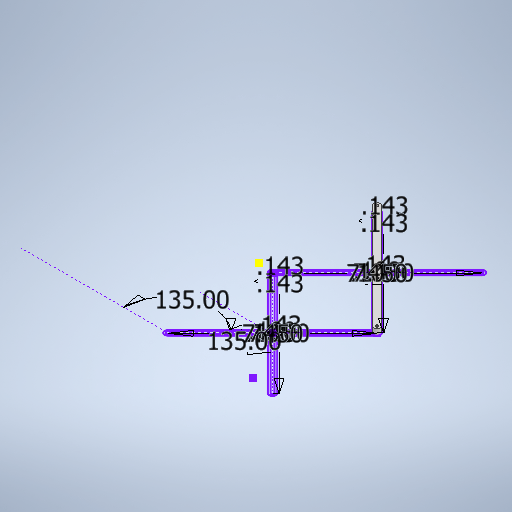
# Autodesk Inventor part: Arm
Saved by Autodesk Inventor 2025.1 (Build 291241000, 241)
## iProperties
Created: 2025-10-25
Part Number: Arm
Material: Generic
Document SubType Name: Modeling
Designer: benja
Density: 1 g/cm^3
Appearance: Default
Author: benja
Autodesk Inventor part; units mm, degrees
ref_plane "YZ Plane" through (0, 0, 0) normal (1, 0, 0) x (0, 1, 0)
ref_plane "XZ Plane" through (0, 0, 0) normal (0, 1, 0) x (-1, 0, 0)
ref_plane "XY Plane" through (0, 0, 0) normal (0, 0, 1) x (1, 0, 0)
sketch "Sketch1" plane through (0, 0, 0) normal (0, 1, 0) x (-1, 0, 0)
  circle A0 centre (-19.4714, 136.4884) radius 1.8097
  line L0 (-19.4714, 136.4884) -> (-153.2772, 2.6825) construction
  line L1 (-20.7511, 137.768) -> (-154.5569, 3.9622)
  line L2 (-151.9975, 1.4028) -> (-18.1917, 135.2087)
  arc A1 (-18.1917, 135.2087) -> (-20.7511, 137.768) centre (-19.4714, 136.4884) ccw
  arc A2 (-154.5569, 3.9622) -> (-151.9975, 1.4028) centre (-153.2772, 2.6825) ccw
  line L3 (-19.4714, 136.4884) -> (169.7586, 136.4884) construction
  line L4 (-87.654, 70.8651) -> (-85.0946, 68.3058)
  line L5 (-87.654, 70.8651) -> (-153.2772, 136.4884)
  line L6 (-87.654, 70.8651) -> (5.1513, 70.8651) construction
  line L7 (-153.2772, 136.4884) -> (-19.4714, 2.6825) construction
  line L8 (-154.5614, 135.2042) -> (-20.7556, 1.3984)
  line L9 (-18.1872, 3.9667) -> (-151.993, 137.7725)
  arc A3 (-151.993, 137.7725) -> (-154.5614, 135.2042) centre (-153.2772, 136.4884) ccw
  arc A4 (-20.7556, 1.3984) -> (-18.1872, 3.9667) centre (-19.4714, 2.6825) ccw
  circle A5 centre (-86.3743, 69.5854) radius 1.8161
  circle A6 centre (-19.4714, 2.6825) radius 1.8161
  line L10 (-150.197, 139.5686) -> (-16.3912, 5.7628)
  arc A7 (-22.5516, -0.3977) -> (-16.3912, 5.7628) centre (-19.4714, 2.6825) ccw
  line L11 (-22.5516, -0.3977) -> (-156.3574, 133.4081)
  arc A8 (-150.197, 139.5686) -> (-156.3574, 133.4081) centre (-153.2772, 136.4884) ccw
  line L12 (-16.3957, 133.4126) -> (-150.2015, -0.3932)
  arc A9 (-156.3529, 5.7583) -> (-150.2015, -0.3932) centre (-153.2772, 2.6825) ccw
  line L13 (-156.3529, 5.7583) -> (-22.5471, 139.5641)
  arc A10 (-16.3957, 133.4126) -> (-22.5471, 139.5641) centre (-19.4714, 136.4884) ccw
  line L14 (-87.654, -62.9407) -> (-85.0946, -65.5001)
  arc A11 (-20.7556, -132.4075) -> (-18.1872, -129.8391) centre (-19.4714, -131.1233) ccw
  circle A12 centre (-19.4714, -131.1233) radius 1.8161
  arc A13 (-22.5516, -134.2035) -> (-16.3912, -128.0431) centre (-19.4714, -131.1233) ccw
  arc A14 (-18.1917, 1.4028) -> (-20.7511, 3.9622) centre (-19.4714, 2.6825) ccw
  arc A15 (-16.3957, -0.3932) -> (-22.5471, 5.7583) centre (-19.4714, 2.6825) ccw
  line L15 (-19.4714, 2.6825) -> (-153.2772, -131.1233) construction
  line L16 (-20.7511, 3.9622) -> (-154.5569, -129.8436)
  line L17 (-151.9975, -132.403) -> (-18.1917, 1.4028)
  arc A16 (-154.5569, -129.8436) -> (-151.9975, -132.403) centre (-153.2772, -131.1233) ccw
  circle A17 centre (-86.3743, -64.2204) radius 1.8161
  arc A18 (-156.3529, -128.0475) -> (-150.2015, -134.199) centre (-153.2772, -131.1233) ccw
  line L18 (-16.3957, -0.3932) -> (-150.2015, -134.199)
  line L19 (-150.197, 5.7628) -> (-16.3912, -128.0431)
  line L20 (-18.1872, -129.8391) -> (-151.993, 3.9667)
  line L21 (-153.2772, 2.6825) -> (-19.4714, -131.1233) construction
  line L22 (-154.5614, 1.3984) -> (-20.7556, -132.4075)
  line L23 (-22.5516, -134.2035) -> (-156.3574, -0.3977)
  line L24 (-156.3529, -128.0475) -> (-22.5471, 5.7583)
  line L25 (-87.654, -62.9407) -> (-153.2772, 2.6825)
  arc A19 (-151.993, 3.9667) -> (-154.5614, 1.3984) centre (-153.2772, 2.6825) ccw
  arc A20 (-150.197, 5.7628) -> (-156.3574, -0.3977) centre (-153.2772, 2.6825) ccw
  circle A21 centre (-153.2772, 2.6825) radius 1.8161
  point P0 (0, 0)
  point P1 (-124.0658, 132.6784)
  point P2 (-86.3743, 69.5854)
  point P3 (-86.3743, -64.2204)
  point P4 (-87.7613, -63.048)
  point P5 (-85.2019, -65.6074)
  point P6 (-84.9873, -65.3928)
  point P7 (-87.5467, -62.8334)
  point P8 (-151.8902, 1.5101)
  point P9 (-154.4496, 4.0695)
  dimension "d0" = 189.23
  dimension "d1" = 135
  dimension "d2" = 135
  dimension "d3" = 189.23
  dimension "d4" = 3.6322
  dimension "d5" = 3.6322
  dimension "d6" = 3.6322
  dimension "d7" = 2.54
  dimension "d8" = 2.54
  dimension "d9" = 189.23
  dimension "d10" = 189.23
  dimension "d11" = 3.6322
  dimension "d12" = 3.6322
  dimension "d13" = 3.6322
  dimension "d14" = 2.54
  dimension "d15" = 2.54
  constraints: 60 end point, 32 point on circle, 22 centre point, 16 tangent, 8 midpoint, 8 parallel, 5 coincident, 2 equal length, 2 horizontal, 1 concentric, 12 other
  measures "d0" distance of L0.start L0.end
  measures "d1" angle of L0 L3
  measures "d2" angle of L6 L5
  measures "d3" distance of L5.end L7.end
  measures "d4" diameter of A4
  measures "d5" diameter of A5
  measures "d6" diameter of A6
  measures "d7" distance between parallel lines of L9 L10
  measures "d8" distance between parallel lines of L2 L12
  measures "d9" distance of L15.start L15.end
  measures "d10" distance of L21.start L21.end
  measures "d11" diameter of A11
  measures "d12" diameter of A17
  measures "d13" diameter of A12
  measures "d14" distance between parallel lines of L20 L19
  measures "d15" distance between parallel lines of L17 L18
extrude "Extrusion1" add sketch "Sketch1" along normal blind 7.62 contours L19 A13 L23 L18 L22 A11 L20 | L18 L20 L17 L19 | A20 L1 A19 L22 A9 L13 | L13 A9 L22 L24 L23 A20 | L19 L24 L20 L12 | L12 L20 L2 L19 | L17 L20 L16 L19 | L20 A12 L22 L18 | L18 L22 L17 A17 L20 | A20 L19 L2 L20 A19 L1 | L19 L16 L20 L24 | L20 L24 L25 L12 | L12 L25 A21 L2 L20 | L17 A17 L20 | L18 L23 L17 L22 | A11 A12 | A19 A21 L2 A2 L1 | L1 A2 L25 A21 A19 | L22 A21 L25 A9 | A9 L25 L24 L22 | L24 L22 L16 L23 | L2 A21 L20 | L20 L16 A17 L25 L24 | A17 L17 | L17 L14 L16 A17 | A17 L16 L20 | L22 A17 L17 | L17 L23 L16 L22 | L24 L25 A17 L16 L22 | A21 L25 L2 | L17 A17 L16 L14 | L16 L25 A17 | L22 L16 A17 | L25 L16 A17
extrude "Extrusion2" cut sketch "Sketch1" along normal blind 7.62 contours A11 A12 | A19 A21 L2 A2 L1 | L17 L14 L16 A17 | L17 A17 L16 L14
body "Solid1"
